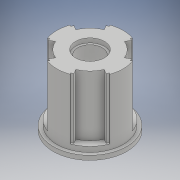
# Autodesk Inventor part: Flanec_pod_diod_N
Saved by Autodesk Inventor 2017 (Build 210142000, 142)
## iProperties
Part Number: Flanec_pod_diod_N
Material: Типовые
Document SubType Name: Modeling
Designer: Тетяна
Density: 1 g/cm^3
Appearance: По умолчанию
Author: Тетяна
Autodesk Inventor part; units mm, degrees
ref_plane "YZ Plane" through (0, 0, 0) normal (1, 0, 0) x (0, 1, 0)
sketch "Эскиз1" plane through (0, 0, 0) normal (0, 1, 0) x (-1, 0, 0)
  circle A0 centre (0, 0) radius 8.4
  dimension "d0" = 16.8
  constraints: 1 centre point, 1 coincident
  measures "d0" diameter of A0
extrude "Выдавливание1" add sketch "Эскиз1" along normal blind 1
sketch "Эскиз2" plane through (0, 1, 0) normal (0, 1, 0) x (1, 0, 0)
  circle A0 centre (0, 0) radius 7.6
  dimension "d3" = 15.2
  constraints: 1 centre point, 1 coincident
  measures "d3" diameter of A0
extrude "Выдавливание2" add sketch "Эскиз2" along normal blind 1.2
sketch "Эскиз3" plane through (0, 2.2, 0) normal (0, 1, 0) x (1, 0, 0)
  circle A0 centre (0, 0) radius 7.6 projected
  line L0 (-7.1372, 2.6117) -> (-2.6117, 7.1372)
  line L1 (-7.1372, 2.6117) -> (-0.7372, 2.6117) construction
  circle A1 centre (0, 0) radius 7.6 projected
  arc A2 (-2.6117, 7.1372) -> (-7.1372, 2.6117) centre (0, 0) ccw
  line L2 (-7.1372, 2.6117) -> (-6.7908, 2.4117)
  line L3 (-7.1372, 2.6117) -> (-6.7372, 2.6117) construction
  line L4 (-4.8744, 4.8744) -> (-7.8113, 7.8113)
  line L5 (-2.6117, 7.1372) -> (-2.4117, 6.7908)
  arc A3 (-2.4117, 6.7908) -> (-6.7908, 2.4117) centre (0, 0) ccw
  line L6 (-6.5909, 2.9139) -> (-2.9139, 6.5909)
  line L7 (-6.5909, 2.9139) -> (-1.3909, 2.9139) construction
  line L8 (-2.9139, 6.5909) -> (-2.3139, 5.5516)
  line L9 (-2.9139, 6.5909) -> (-1.7139, 6.5909) construction
  line L10 (-6.5909, 2.9139) -> (-5.5516, 2.3139)
  arc A4 (-2.3139, 5.5516) -> (-5.5516, 2.3139) centre (0, 0) ccw
  line L11 (-2.6117, -7.1372) -> (-2.4117, -6.7908)
  arc A5 (-7.1372, -2.6117) -> (-2.6117, -7.1372) centre (0, 0) ccw
  line L12 (-7.1372, -2.6117) -> (-6.7908, -2.4117)
  arc A6 (-6.7908, -2.4117) -> (-2.4117, -6.7908) centre (0, 0) ccw
  line L13 (-6.5909, -2.9139) -> (-5.5516, -2.3139)
  arc A7 (-5.5516, -2.3139) -> (-2.3139, -5.5516) centre (0, 0) ccw
  line L14 (-2.9139, -6.5909) -> (-2.3139, -5.5516)
  line L15 (7.1372, -2.6117) -> (6.7908, -2.4117)
  arc A8 (2.6117, -7.1372) -> (7.1372, -2.6117) centre (0, 0) ccw
  line L16 (2.6117, -7.1372) -> (2.4117, -6.7908)
  arc A9 (2.4117, -6.7908) -> (6.7908, -2.4117) centre (0, 0) ccw
  line L17 (2.9139, -6.5909) -> (2.3139, -5.5516)
  arc A10 (2.3139, -5.5516) -> (5.5516, -2.3139) centre (0, 0) ccw
  line L18 (6.5909, -2.9139) -> (5.5516, -2.3139)
  line L19 (2.6117, 7.1372) -> (2.4117, 6.7908)
  arc A11 (7.1372, 2.6117) -> (2.6117, 7.1372) centre (0, 0) ccw
  line L20 (7.1372, 2.6117) -> (6.7908, 2.4117)
  arc A12 (6.7908, 2.4117) -> (2.4117, 6.7908) centre (0, 0) ccw
  line L21 (6.5909, 2.9139) -> (5.5516, 2.3139)
  arc A13 (5.5516, 2.3139) -> (2.3139, 5.5516) centre (0, 0) ccw
  line L22 (2.9139, 6.5909) -> (2.3139, 5.5516)
  dimension "d6" = 6.4
  dimension "d7" = 45
  dimension "d8" = 0.4
  dimension "d9" = 30
  dimension "d10" = 5.2
  dimension "d11" = 45
  dimension "d12" = 1.2
  dimension "d13" = 60
  dimension "d14" = 5.1996
  dimension "d17" = 360
  constraints: 46 end point, 34 point on circle, 12 centre point, 6 coincident, 4 equal length, 4 horizontal, 2 symmetric about line, 1 concentric, 1 midpoint, 71 other
  measures "d6" distance of L0.start L0.end
  measures "d7" angle of L1 L0
  measures "d8" distance of L0.start L2.end
  measures "d9" angle of L2 L3
  measures "d10" distance of L6.start L6.end
  measures "d11" angle of L7 L6
  measures "d12" distance of L6.end L8.end
  measures "d13" angle of L8 L9
  measures "d14" distance from line of L4.end L1
extrude "Выдавливание3" add sketch "Эскиз3" along normal blind 13.8 separate body contours L20 A12 L19 A0 | A0 L16 A9 L15 | L0 A3 L4 A0 | L5 A3 L0 | L21 A13 L22 A12 | A0 L12 A6 L11 | A9 L17 A10 L18 | L4 A3 L0 A0 | A3 L6 L0 | L0 L4 A3 | L0 A3 L2 | L4 L0 A3 | L8 A4 L10 L6 | A6 L13 A7 L14
sketch "Эскиз4" plane through (0, 2.2, 0) normal (0, 1, 0) x (1, 0, 0)
  circle A0 centre (0, 0) radius 7.6 projected
extrude "Выдавливание4" add sketch "Эскиз4" along normal up to surface (13.8 mm away) bodies 1
combine bodies "Комбинировать1" operation type subtract main body 1 bodies to subtract 2
sketch "Эскиз5" plane through (0, 1, 0) normal (0, 1, 0) x (1, 0, 0)
  arc A0 (5.5516, 2.3139) -> (2.3139, 5.5516) centre (0, 0) ccw projected
  circle A1 centre (0, 0) radius 6
  dimension "d23" = 12
  constraints: 1 centre point, 1 coincident
  measures "d23" diameter of A1
ref_plane "РабПлоскость1" through (0, 11, 0) normal (0, 1, 0) x (1, 0, 0)
sketch "Эскиз6" plane through (0, 11, 0) normal (0, 1, 0) x (1, 0, 0)
  circle A0 centre (0, 0) radius 2.9
  dimension "d25" = 5.8
  constraints: 1 centre point, 1 coincident
  measures "d25" diameter of A0
sketch "Эскиз7" plane through (0, 0, 0) normal (0, 0, 1) x (1, 0, 0)
  line L0 (2.9, 11) -> (-2.9, 11) projected
  line L1 (6, 1) -> (-6, 1) projected
  line L2 (2.9, 11) -> (6, 1)
  line L3 (0, 11) -> (0, 1)
  point P0 (0, 0)
  constraints: 4 end point, 2 midpoint
revolve "Вращение1" add sketch "Эскиз7" angle 360 about axis through (0, 11, 0) along (0, -1, 0) separate body
combine bodies "Комбинировать2" operation type subtract main body 1 bodies to subtract 3
sketch "Эскиз8" plane through (0, 16, 0) normal (0, 1, 0) x (1, 0, 0)
  arc A0 (7.1372, 2.6117) -> (7.1372, -2.6117) centre (0, 0) ccw projected
  circle A1 centre (0, 0) radius 2.8
  dimension "d27" = 5.6
  constraints: 1 centre point, 1 coincident
  measures "d27" diameter of A1
extrude "Выдавливание5" cut sketch "Эскиз8" against normal blind 5 bodies 1
sketch "Эскиз9" plane through (0, 16, 0) normal (0, 1, 0) x (1, 0, 0)
  circle A0 centre (0, 0) radius 2.8 projected
  arc A1 (7.1372, 2.6117) -> (7.1372, -2.6117) centre (0, 0) ccw projected
  circle A2 centre (0, 0) radius 3.3
  dimension "d30" = 6.6
  constraints: 1 centre point, 1 coincident
  measures "d30" diameter of A2
extrude "Выдавливание6" cut sketch "Эскиз9" against normal blind 1 bodies 1
ref_plane "РабПлоскость2" through (-4.2529, 2.2, -4.2529) normal (0.7071068, 0, 0.7071068) x (0, 1, 0)
